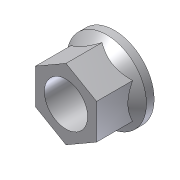
# Autodesk Inventor part: MS21042-04
Saved by Autodesk Inventor 2014 SP1 (Build 180222100, 222)
## iProperties
Created: 2009-09-16
Part Number: MS21042-04
Document SubType Name: Modeling
Designer: Robert Davis
Density: 1 g/cm^3
Description: LOCKING NUT, #4-40
Mass: 0.0298518 g
Surface Area: 1.00229 cm^2
Volume: 0.0298518 cm^3
Material: Generic
Appearance: Default
Author: Robert Davis
Autodesk Inventor part; units mm, degrees
ref_plane "YZ Plane" through (0, 0, 0) normal (1, 0, 0) x (0, 1, 0)
ref_plane "XZ Plane" through (0, 0, 0) normal (0, 1, 0) x (-1, 0, 0)
ref_plane "XY Plane" through (0, 0, 0) normal (0, 0, 1) x (1, 0, 0)
sketch "Sketch1" plane through (0, 0, 0) normal (0, 0, 1) x (1, 0, 0)
  circle A0 centre (0, 0) radius 2.6162
  dimension "d0" = 5.2324
  constraints: 1 centre point
  measures "d0" diameter of A0
extrude "Extrusion1" add sketch "Sketch1" along normal blind 0.508
sketch "Sketch2" plane through (0, 0, 0.508) normal (0, 0, 1) x (1, 0, 0)
  circle A0 centre (0, 0) radius 2.6162 projected
  circle A1 centre (0, 0) radius 2.6162
  constraints: 1 centre point, 1 coincident, 1 concentric
extrude "Extrusion2" add sketch "Sketch2" along normal blind 2.54 draft -45
sketch "Sketch3" plane through (0, 0, 0) normal (0, 0, -1) x (-1, 0, 0)
  circle A0 centre (0, 0) radius 2.6162 projected
  line L0 (-2.0066, 1.1585) -> (0, 2.317)
  line L1 (0, 2.317) -> (2.0066, 1.1585)
  line L2 (2.0066, 1.1585) -> (2.0066, -1.1585)
  line L3 (2.0066, -1.1585) -> (0, -2.317)
  line L4 (0, -2.317) -> (-2.0066, -1.1585)
  line L5 (-2.0066, -1.1585) -> (-2.0066, 1.1585)
  dimension "d5" = 4.0132
  constraints: 12 end point, 1 coincident, 13 other
  measures "d5" distance between parallel lines of L2 L5
extrude "Extrusion3" add sketch "Sketch3" against normal blind 3.175 contours L0 L1 L2 L3 L4 L5
sketch "Sketch4" plane through (0, 0, 0) normal (0, 0, -1) x (-1, 0, 0)
  circle A0 centre (0, 0) radius 2.6162 projected
  circle A1 centre (0, 0) radius 1.4224
  dimension "d8" = 2.8448
  constraints: 1 centre point, 1 coincident
  measures "d8" diameter of A1
extrude "Extrusion4" cut sketch "Sketch4" against normal through all contours A1
body "Solid1"
